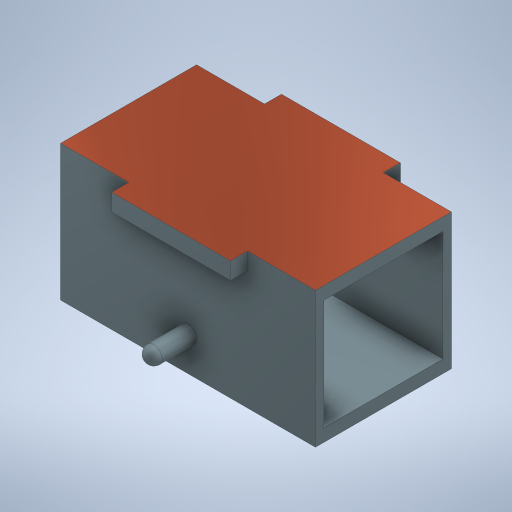
# Autodesk Inventor part: Battery Container
Saved by Autodesk Inventor 2023 (Build 270158000, 158)
## iProperties
Created: 2022-10-27
Part Number: Battery Container
Material: Iron, Malleable
Document SubType Name: Modeling
Designer: cheng
Density: 7.15 g/cm^3
Appearance: Lead
Author: cheng
Autodesk Inventor part; units mm, degrees
ref_plane "YZ Plane" through (0, 0, 0) normal (1, 0, 0) x (0, 1, 0)
ref_plane "XZ Plane" through (0, 0, 0) normal (0, 1, 0) x (-1, 0, 0)
ref_plane "XY Plane" through (0, 0, 0) normal (0, 0, 1) x (1, 0, 0)
sketch "Sketch1" plane through (0, 0, 0) normal (0, 1, 0) x (-1, 0, 0)
  line L0 (75, -40) -> (-75, -40)
  line L1 (-75, -40) -> (-75, 40)
  line L2 (-75, 40) -> (75, 40)
  line L3 (75, 40) -> (75, -40)
  line L4 (75, -40) -> (-75, 40) construction
  line L5 (-75, -40) -> (75, 40) construction
  point P0 (0, 0)
  dimension "d0" = 80
  dimension "d1" = 150
  constraints: 12 end point, 2 midpoint, 2 parallel, 1 horizontal, 1 perpendicular
  measures "d0" distance of L0.end L1.end
  measures "d1" distance of L0.start L0.end
extrude "Extrusion1" add sketch "Sketch1" along normal blind 80
sketch "Sketch2" plane through (75, 0, 40) normal (1, 0, 0) x (0, 0, -1)
  line L0 (0, 0) -> (0, 80) projected
  line L1 (0, 40) -> (80, 40)
  line L2 (80, 0) -> (80, 80) projected
  line L3 (40, 0) -> (40, 80)
  line L4 (0, 80) -> (80, 80) projected
  line L5 (75, 72.5) -> (5, 72.5)
  line L6 (5, 72.5) -> (5, 7.5)
  line L7 (5, 7.5) -> (75, 7.5)
  line L8 (75, 7.5) -> (75, 72.5)
  line L9 (75, 72.5) -> (5, 7.5) construction
  line L10 (5, 72.5) -> (75, 7.5) construction
  point P0 (40, 40)
  dimension "d4" = 70
  dimension "d5" = 65
  constraints: 16 end point, 6 midpoint, 2 parallel, 1 horizontal, 1 perpendicular
  measures "d4" distance between parallel lines of L8 L6
  measures "d5" distance between parallel lines of L5 L7
extrude "Extrusion2" cut sketch "Sketch2" against normal blind 143.6625 contours L6 L5 L3 L1 | L1 L3 L7 L6 | L3 L5 L8 L1 | L1 L8 L7 L3
sketch "Sketch3" plane through (-75, 0, 40) normal (0, 0, 1) x (1, 0, 0)
  line L0 (75, 0) -> (75, 49.7289)
  line L1 (110, 80) -> (40, 80)
  line L2 (40, 80) -> (40, 70)
  line L3 (40, 70) -> (110, 70)
  line L4 (110, 70) -> (110, 80)
  line L5 (110, 80) -> (40, 70) construction
  line L6 (40, 80) -> (110, 70) construction
  line L7 (0, 80) -> (150, 80) projected
  point P0 (75, 75)
  dimension "d8" = 70
  dimension "d9" = 10
  dimension "d17" = 0
  constraints: 14 end point, 2 midpoint, 2 parallel, 1 horizontal, 1 perpendicular, 1 point on line, 1 vertical
  measures "d8" distance of L1.start L1.end
  measures "d9" distance of L3.end L1.start
  measures "d17" distance between parallel lines of L1 L7
extrude "Extrusion3" add sketch "Sketch3" along normal blind 10
sketch "Sketch5" plane through (75, 0, -40) normal (0, 0, -1) x (-1, 0, 0)
  line L0 (75, 0) -> (75, 49.9117)
  line L1 (110, 80) -> (40, 80)
  line L2 (40, 80) -> (40, 70)
  line L3 (40, 70) -> (110, 70)
  line L4 (110, 70) -> (110, 80)
  line L5 (110, 80) -> (40, 70) construction
  line L6 (40, 80) -> (110, 70) construction
  line L7 (0, 80) -> (150, 80) projected
  point P0 (75, 75)
  dimension "d12" = 70
  dimension "d13" = 10
  dimension "d14" = 0
  constraints: 14 end point, 2 midpoint, 2 parallel, 1 horizontal, 1 perpendicular, 1 point on line, 1 vertical
  measures "d12" distance of L1.start L1.end
  measures "d13" distance of L3.end L1.start
  measures "d14" distance between parallel lines of L7 L1
extrude "Extrusion4" add sketch "Sketch5" along normal blind 10
sketch "Sketch8" plane through (-75, 0, 40) normal (0, 0, 1) x (1, 0, 0)
  line L0 (0, 0) -> (0, 80) projected
  line L1 (0, 40) -> (75, 40) construction
  line L2 (75, 40) -> (75, 0) construction
  line L3 (0, 20) -> (75, 20) construction
  circle A0 centre (75, 20) radius 5
  dimension "d24" = 10
  constraints: 6 end point, 2 midpoint, 1 centre point, 1 coincident, 1 horizontal, 1 parallel, 1 perpendicular, 1 point on line
  measures "d24" diameter of A0
extrude "Extrusion5" add sketch "Sketch8" along normal blind 25
sketch "Sketch9" plane through (75, 0, -40) normal (0, 0, -1) x (-1, 0, 0)
  line L0 (0, 0) -> (0, 80) projected
  line L1 (0, 40) -> (75, 40) construction
  line L2 (75, 40) -> (75, 0) construction
  circle A0 centre (75, 20) radius 5 projected
  line L3 (0, 20) -> (75, 20) construction
  circle A1 centre (75, 20) radius 5
  dimension "d25" = 10
  constraints: 6 end point, 2 horizontal, 1 centre point, 1 coincident, 1 midpoint, 1 perpendicular, 1 point on line
  measures "d25" diameter of A1
extrude "Extrusion6" add sketch "Sketch9" along normal blind 25
fillet "Fillet1" radius 4.7625 1 edges at (-5, 20, 65)
fillet "Fillet2" radius 4.7625 1 edges at (5, 20, -65)
body "Solid1"
